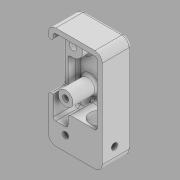
# Autodesk Inventor part: case
Saved by Autodesk Inventor 2020 (Build 240168000, 168)
## iProperties
Created: 2019-10-12
Part Number: case
Material: Generic
Document SubType Name: Modeling
Designer: ROBERTO
Density: 1 g/cm^3
Appearance: Default
Author: gera
Autodesk Inventor part; units mm, degrees
ref_plane "YZ Plane" through (0, 0, 0) normal (1, 0, 0) x (0, 1, 0)
ref_plane "XZ Plane" through (0, 0, 0) normal (0, 1, 0) x (-1, 0, 0)
ref_plane "XY Plane" through (0, 0, 0) normal (0, 0, 1) x (1, 0, 0)
sketch "Sketch1" plane through (0, 0, 0) normal (0, 0, 1) x (1, 0, 0)
  line L0 (9.525, 16.232681) -> (60.325, 16.232681) construction
  line L1 (9.525, 6.707681) -> (60.325, 6.707681)
  arc A0 (0, 16.232681) -> (9.525, 6.707681) centre (9.525, 16.232681) ccw
  arc A1 (60.325, 6.707681) -> (69.85, 16.232681) centre (60.325, 16.232681) ccw
  line L2 (9.525, 130.532681) -> (60.325, 130.532681) construction
  line L3 (60.325, 140.057681) -> (9.525, 140.057681)
  arc A2 (9.525, 140.057681) -> (0, 130.532681) centre (9.525, 130.532681) ccw
  arc A3 (69.85, 130.532681) -> (60.325, 140.057681) centre (60.325, 130.532681) ccw
  line L4 (69.85, 130.532681) -> (69.85, 16.232681)
  line L5 (0, 130.532681) -> (0, 16.232681)
  line L6 (0, -28.406075) -> (0, 170.436448) construction
  point P0 (0, 0)
  point P1 (34.925, 16.232681)
  point P2 (34.925, 130.532681)
  dimension "d0" = 133.35
  dimension "d1" = 69.85
  dimension "d2" = 9.525
  constraints: 16 end point, 8 point on circle, 8 tangent, 4 centre point, 3 equal radius, 2 midpoint, 2 vertical, 1 collinear, 1 horizontal, 1 point on line
  measures "d0" distance between parallel lines of L1 L3
  measures "d1" distance between parallel lines of L4 L5
  measures "d2" radius of A3
extrude "Extrusion1" add sketch "Sketch1" along normal blind 38.1
sketch "Sketch2" plane through (0, 0, 38.1) normal (0, 0, 1) x (1, 0, 0)
  arc A0 (69.85, 130.532681) -> (60.325, 140.057681) centre (60.325, 130.532681) ccw construction
  line L0 (60.325, 140.057681) -> (9.525, 140.057681) construction
  arc A1 (9.525, 140.057681) -> (0, 130.532681) centre (9.525, 130.532681) ccw construction
  line L1 (0, 130.532681) -> (0, 16.232681) construction
  arc A2 (0, 16.232681) -> (9.525, 6.707681) centre (9.525, 16.232681) ccw construction
  line L2 (9.525, 6.707681) -> (60.325, 6.707681) construction
  arc A3 (60.325, 6.707681) -> (69.85, 16.232681) centre (60.325, 16.232681) ccw construction
  line L3 (69.85, 16.232681) -> (69.85, 130.532681) construction
  arc A4 (9.525, 133.707681) -> (6.35, 130.532681) centre (9.525, 130.532681) ccw
  arc A5 (63.5, 130.532681) -> (60.325, 133.707681) centre (60.325, 130.532681) ccw
  arc A6 (60.325, 51.157681) -> (63.5, 54.332681) centre (60.325, 54.332681) ccw
  arc A7 (22.225, 35.282681) -> (25.4, 38.457681) centre (22.225, 38.457681) ccw
  arc A8 (6.35, 38.457681) -> (9.525, 35.282681) centre (9.525, 38.457681) ccw
  line L4 (9.525, 133.707681) -> (61.946324, 133.707681)
  line L5 (6.35, 132.10409) -> (6.35, 35.282681)
  line L6 (63.5, 133.707681) -> (63.5, 54.332681)
  line L7 (69.85, 16.232681) -> (69.85, 130.532681)
  line L8 (6.35, 35.282681) -> (22.225, 35.282681)
  line L9 (25.4, 38.457681) -> (25.4, 50.542115)
  line L10 (60.325, 51.157681) -> (28.575, 51.157681)
  arc A9 (28.575, 51.157681) -> (25.4, 47.982681) centre (28.575, 47.982681) ccw
  point P0 (0, 0)
  dimension "d5" = 6.35
  dimension "d6" = 6.35
  dimension "d7" = 38.1
  dimension "d8" = 15.875
  dimension "d9" = 44.45
  constraints: 12 end point, 12 point on circle, 11 tangent, 6 centre point, 6 point on line, 5 equal radius, 2 coincident, 2 horizontal, 2 vertical, 1 parallel, 1 perpendicular
  measures "d5" distance between parallel lines of L0 L4
  measures "d6" distance between parallel lines of L5 L1
  measures "d7" distance between parallel lines of L6 L9
  measures "d8" distance between parallel lines of L10 L8
  measures "d9" distance between parallel lines of L2 L10
extrude "Extrusion2" cut sketch "Sketch2" against normal blind 31.75 contours L4 A5 L6 A6 L10 A9 L9 A7 L8 A8 L5 A4
sketch "Sketch3" plane through (0, 16.232681, 0) normal (-1, 0, 0) x (0, 0, 1)
  line L0 (0, 114.3) -> (0, 0) construction
  line L1 (0, 0) -> (38.1, 0) construction
  line L2 (38.1, 114.3) -> (38.1, 0) construction
  line L3 (0, 114.3) -> (38.1, 114.3) construction
  line L4 (38.1, 107.95) -> (20.6375, 107.95)
  line L5 (19.05, 106.3625) -> (19.05, 49.2125)
  line L6 (20.6375, 47.625) -> (38.1, 47.625)
  line L7 (38.1, 47.625) -> (38.1, 107.95)
  arc A0 (20.6375, 107.95) -> (19.05, 106.3625) centre (20.6375, 106.3625) ccw
  arc A1 (19.05, 49.2125) -> (20.6375, 47.625) centre (20.6375, 49.2125) ccw
  line L8 (0, 123.825) -> (38.1, 123.825) projected
  point P0 (0, -16.232681)
  dimension "d12" = 19.05
  dimension "d13" = 60.325
  dimension "d14" = 15.875
  dimension "d15" = 3.175
  constraints: 8 end point, 4 point on circle, 4 tangent, 2 centre point, 2 parallel, 1 collinear, 1 equal radius, 1 horizontal, 1 perpendicular
  measures "d12" distance between parallel lines of L5 L2
  measures "d13" distance between parallel lines of L6 L4
  measures "d14" distance between parallel lines of L4 L8
  measures "d15" diameter of A0
extrude "Extrusion3" cut sketch "Sketch3" against normal blind 6.35
sketch "Sketch4" plane through (0, 0, 6.35) normal (0, 0, 1) x (1, 0, 0)
  line L0 (25.4, 47.982681) -> (25.4, 38.457681) construction
  arc A0 (28.575, 51.157681) -> (25.4, 47.982681) centre (28.575, 47.982681) ccw construction
  line L1 (60.325, 51.157681) -> (28.575, 51.157681) construction
  arc A1 (60.325, 51.157681) -> (63.5, 54.332681) centre (60.325, 54.332681) ccw construction
  line L2 (63.5, 130.532681) -> (63.5, 54.332681) construction
  arc A2 (63.5, 130.532681) -> (60.325, 133.707681) centre (60.325, 130.532681) ccw construction
  line L3 (9.525, 133.707681) -> (60.325, 133.707681) construction
  arc A3 (9.525, 133.707681) -> (6.35, 130.532681) centre (9.525, 130.532681) ccw construction
  line L4 (6.35, 38.457681) -> (6.35, 130.532681) construction
  arc A4 (6.35, 38.457681) -> (9.525, 35.282681) centre (9.525, 38.457681) ccw construction
  line L5 (22.225, 35.282681) -> (9.525, 35.282681) construction
  arc A5 (22.225, 35.282681) -> (25.4, 38.457681) centre (22.225, 38.457681) ccw construction
  line L6 (0, 65.445181) -> (0, 122.595181) construction
  line L7 (0, 65.445181) -> (0, 122.595181) construction
  line L8 (0, 65.445181) -> (6.35, 65.445181) construction
  line L9 (6.35, 122.595181) -> (6.35, 65.445181) construction
  line L10 (0, 122.595181) -> (6.35, 122.595181) construction
  line L11 (6.35, 63.857681) -> (0, 63.857681) construction
  line L12 (0, 63.857681) -> (0, 16.232681) construction
  arc A6 (0, 16.232681) -> (9.525, 6.707681) centre (9.525, 16.232681) ccw construction
  line L13 (9.525, 6.707681) -> (60.325, 6.707681) construction
  arc A7 (60.325, 6.707681) -> (69.85, 16.232681) centre (60.325, 16.232681) ccw construction
  line L14 (69.85, 16.232681) -> (69.85, 130.532681) construction
  arc A8 (69.85, 130.532681) -> (60.325, 140.057681) centre (60.325, 130.532681) ccw construction
  line L15 (60.325, 140.057681) -> (9.525, 140.057681) construction
  arc A9 (9.525, 140.057681) -> (0, 130.532681) centre (9.525, 130.532681) ccw construction
  line L16 (0, 130.532681) -> (0, 124.182681) construction
  line L17 (0, 124.182681) -> (6.35, 124.182681) construction
  line L18 (6.35, 124.182681) -> (6.35, 130.532681) construction
  arc A10 (9.525, 133.707681) -> (6.35, 130.532681) centre (9.525, 130.532681) ccw construction
  line L19 (9.525, 133.707681) -> (60.325, 133.707681) construction
  arc A11 (63.5, 130.532681) -> (60.325, 133.707681) centre (60.325, 130.532681) ccw construction
  line L20 (63.5, 130.532681) -> (63.5, 54.332681) construction
  arc A12 (60.325, 51.157681) -> (63.5, 54.332681) centre (60.325, 54.332681) ccw construction
  line L21 (60.325, 51.157681) -> (28.575, 51.157681) construction
  arc A13 (28.575, 51.157681) -> (25.4, 47.982681) centre (28.575, 47.982681) ccw construction
  line L22 (25.4, 47.982681) -> (25.4, 38.457681) construction
  arc A14 (22.225, 35.282681) -> (25.4, 38.457681) centre (22.225, 38.457681) ccw construction
  line L23 (22.225, 35.282681) -> (9.525, 35.282681) construction
  arc A15 (6.35, 38.457681) -> (9.525, 35.282681) centre (9.525, 38.457681) ccw construction
  line L24 (6.35, 38.457681) -> (6.35, 63.857681) construction
  line L25 (0, 124.182681) -> (6.35, 124.182681)
  line L26 (6.35, 124.182681) -> (12.7, 124.182681)
  line L27 (12.7, 98.782681) -> (6.35, 98.782681)
  line L28 (6.35, 124.182681) -> (6.35, 98.782681)
  line L29 (6.35, 38.457681) -> (6.35, 130.532681)
  arc A16 (6.35, 122.481204) -> (5.46153, 121.917936) centre (12.7, 111.482681) ccw
  arc A17 (12.7, 98.782681) -> (12.7, 124.182681) centre (12.7, 111.482681) ccw
  point P0 (0, 0)
  dimension "d19" = 104.775
  dimension "d20" = 12.7
  constraints: 6 end point, 5 point on circle, 2 centre point, 2 point on line, 1 horizontal, 1 tangent, 3 other
  measures "d19" distance from line of L13 A16.centre
  measures "d20" distance from line of A16.centre L6
extrude "Extrusion4" add sketch "Sketch4" along normal blind 12.7
sketch "Sketch5" plane through (0, 0, 6.35) normal (0, 0, 1) x (1, 0, 0)
  circle A0 centre (22.225, 67.032681) radius 9.525
  line L0 (6.35, 63.857681) -> (0, 63.857681) construction
  line L1 (0, 63.857681) -> (0, 16.232681) construction
  arc A1 (0, 16.232681) -> (9.525, 6.707681) centre (9.525, 16.232681) ccw construction
  line L2 (9.525, 6.707681) -> (60.325, 6.707681) construction
  arc A2 (60.325, 6.707681) -> (69.85, 16.232681) centre (60.325, 16.232681) ccw construction
  line L3 (69.85, 16.232681) -> (69.85, 130.532681) construction
  arc A3 (69.85, 130.532681) -> (60.325, 140.057681) centre (60.325, 130.532681) ccw construction
  line L4 (60.325, 140.057681) -> (9.525, 140.057681) construction
  arc A4 (9.525, 140.057681) -> (0, 130.532681) centre (9.525, 130.532681) ccw construction
  line L5 (0, 130.532681) -> (0, 124.182681) construction
  line L6 (0, 124.182681) -> (6.35, 124.182681) construction
  line L7 (6.35, 124.182681) -> (6.35, 130.532681) construction
  arc A5 (9.525, 133.707681) -> (6.35, 130.532681) centre (9.525, 130.532681) ccw construction
  line L8 (9.525, 133.707681) -> (60.325, 133.707681) construction
  arc A6 (63.5, 130.532681) -> (60.325, 133.707681) centre (60.325, 130.532681) ccw construction
  line L9 (63.5, 130.532681) -> (63.5, 54.332681) construction
  arc A7 (60.325, 51.157681) -> (63.5, 54.332681) centre (60.325, 54.332681) ccw construction
  line L10 (60.325, 51.157681) -> (28.575, 51.157681) construction
  arc A8 (28.575, 51.157681) -> (25.4, 47.982681) centre (28.575, 47.982681) ccw construction
  line L11 (25.4, 47.982681) -> (25.4, 38.457681) construction
  arc A9 (22.225, 35.282681) -> (25.4, 38.457681) centre (22.225, 38.457681) ccw construction
  line L12 (22.225, 35.282681) -> (9.525, 35.282681) construction
  arc A10 (6.35, 38.457681) -> (9.525, 35.282681) centre (9.525, 38.457681) ccw construction
  line L13 (6.35, 38.457681) -> (6.35, 63.857681) construction
  line L14 (6.35, 124.182681) -> (12.7, 124.182681) construction
  arc A11 (12.7, 98.782681) -> (12.7, 124.182681) centre (12.7, 111.482681) ccw construction
  line L15 (12.7, 98.782681) -> (6.35, 98.782681) construction
  line L16 (6.35, 38.457681) -> (6.35, 98.782681) construction
  arc A12 (6.35, 38.457681) -> (9.525, 35.282681) centre (9.525, 38.457681) ccw construction
  line L17 (22.225, 35.282681) -> (9.525, 35.282681) construction
  arc A13 (22.225, 35.282681) -> (25.4, 38.457681) centre (22.225, 38.457681) ccw construction
  line L18 (25.4, 47.982681) -> (25.4, 38.457681) construction
  arc A14 (28.575, 51.157681) -> (25.4, 47.982681) centre (28.575, 47.982681) ccw construction
  line L19 (60.325, 51.157681) -> (28.575, 51.157681) construction
  arc A15 (60.325, 51.157681) -> (63.5, 54.332681) centre (60.325, 54.332681) ccw construction
  line L20 (63.5, 130.532681) -> (63.5, 54.332681) construction
  arc A16 (63.5, 130.532681) -> (60.325, 133.707681) centre (60.325, 130.532681) ccw construction
  line L21 (9.525, 133.707681) -> (60.325, 133.707681) construction
  arc A17 (9.525, 133.707681) -> (6.35, 130.532681) centre (9.525, 130.532681) ccw construction
  line L22 (6.35, 124.182681) -> (6.35, 130.532681) construction
  point P0 (0, 0)
  dimension "d25" = 19.05
  dimension "d26" = 60.325
  dimension "d27" = 22.225
  constraints: 1 centre point
  measures "d25" diameter of A0
  measures "d26" distance from line of L2 A0.centre
  measures "d27" distance from line of L1 A0.centre
extrude "Extrusion5" add sketch "Sketch5" along normal blind 31.75
sketch "Sketch6" plane through (9.525, 6.707681, 0) normal (0, -1, 0) x (1, 0, 0)
  line L0 (60.325, 0) -> (60.325, 38.1) construction
  line L1 (0, 38.1) -> (50.8, 38.1) construction
  point P0 (-9.525, 0)
  point P1 (41.275, 22.225)
  dimension "d30" = 19.05
  dimension "d31" = 15.875
  measures "d30" distance from line of L0 point (41.275, 22.225)
  measures "d31" distance from line of L1 point (41.275, 22.225)
hole "Hole1" at (50.8, 6.707681, 22.225) direction (0, 1, 0) diameter 25.4 depth 44.45 tip angle 118
fillet "Fillet1" radius 3.175 15 edges at (12.7, 67.0327, 6.35) (7.2799, 36.2126, 6.35) (15.875, 35.2827, 6.35) (24.4701, 36.2126, 6.35) (25.4, 43.2202, 6.35) (26.3299, 50.2277, 6.35) (44.45, 51.1577, 6.35) (62.5701, 52.0876, 6.35) (63.5, 92.4327, 6.35) (62.5701, 132.7777, 6.35) (34.925, 133.7077, 6.35) (7.2799, 132.7777, 6.35) (6.35, 127.3577, 6.35) (6.35, 68.6202, 6.35) (6.35, 124.1827, 12.7)
fillet "Fillet2" radius 3.175 6 edges at (11.1124, 98.7827, 6.35) (7.2799, 98.7827, 7.2799) (6.35, 98.7827, 14.2875) (11.1124, 124.1827, 6.35) (7.2799, 125.1126, 7.2799) (25.4, 111.4827, 6.35)
fillet "Fillet3" radius 3.175 7 edges at (0, 64.3226, 19.515) (0, 94.0202, 19.05) (0, 123.7177, 19.515) (0, 124.1827, 29.3687) (0, 63.8577, 29.3688) (6.35, 124.1827, 29.3687) (6.35, 123.7177, 19.515)
fillet "Fillet4" radius 3.175 8 edges at (67.0602, 9.4975, 0) (69.85, 73.3827, 0) (67.0602, 137.2679, 0) (34.925, 140.0577, 0) (2.7898, 137.2679, 0) (0, 73.3827, 0) (2.7898, 9.4975, 0) (34.925, 6.7077, 0)
sketch "Sketch7" plane through (12.7, 111.482681, 19.05) normal (0, 0, 1) x (1, 0, 0)
  line L0 (-9.525, -46.0375) -> (-9.525, 11.1125) construction
  line L1 (-9.525, -46.0375) -> (-6.35, -46.0375) construction
  line L2 (-6.35, -15.875) -> (-6.35, -46.0375) construction
  arc A0 (-3.175, -12.7) -> (-6.35, -15.875) centre (-3.175, -15.875) ccw construction
  line L3 (-3.175, -12.7) -> (0, -12.7) construction
  arc A1 (0, -12.7) -> (0, 12.7) centre (0, 0) ccw construction
  line L4 (0, 12.7) -> (-3.175, 12.7) construction
  arc A2 (-6.35, 15.875) -> (-3.175, 12.7) centre (-3.175, 15.875) ccw construction
  line L5 (-6.35, 15.602628) -> (-6.35, 15.875) construction
  arc A3 (0, -12.7) -> (0, 12.7) centre (0, 0) ccw construction
  point P0 (-12.7, -111.482681)
  constraints: 1 coincident, 1 other
hole "Hole2" at (12.7, 111.482681, 19.05) direction (0, 0, -1) diameter 9.525 end through all
sketch "Sketch11" plane through (69.85, 16.232681, 38.1) normal (1, 0, 0) x (0, 0, -1)
  line L0 (0, 0) -> (0, 114.3)
  line L1 (34.925, -9.525) -> (24.27526, -9.525)
  point P0 (38.1, -16.232681)
  point P1 (15.875, 12.7)
  dimension "d75" = 15.875
  dimension "d76" = 22.225
  measures "d75" distance from line of L0 point (15.875, 12.7)
  measures "d76" distance from line of L1 point (15.875, 12.7)
hole "Hole6" at (69.85, 28.932681, 22.225) direction (-1, 0, 0) diameter 7.9375 depth 15.24
sketch "Sketch12" plane through (0, 0, 0) normal (0, 0, -1) x (-1, 0, 0)
  line L0 (0, 16.232681) -> (0, 130.532681)
  line L1 (-60.325, 6.707681) -> (-9.525, 6.707681)
  point P0 (0, 0)
  point P1 (-22.225, 67.032681)
  dimension "d86" = 22.225
  dimension "d87" = 60.325
  measures "d86" distance from line of L0 point (-22.225, 67.033)
  measures "d87" distance from line of L1 point (-22.225, 67.033)
hole "Hole7" at (22.225, 67.032681, 0) direction (0, 0, 1) diameter 7.9375 end through all counterbore diameter 12.7 counterbore depth 7.9375
sketch "Sketch13" plane through (0, 0, 0) normal (0, 0, -1) x (-1, 0, 0)
  line L0 (0, 16.232681) -> (0, 130.532681)
  line L1 (-60.325, 6.707681) -> (-9.525, 6.707681)
  point P0 (0, 0)
  point P1 (-22.225, 25.757681)
  dimension "d95" = 22.225
  dimension "d96" = 19.05
  measures "d95" distance from line of L0 point (-22.225, 25.758)
  measures "d96" distance from line of L1 point (-22.225, 25.758)
hole "Hole8" at (22.225, 25.757681, 0) direction (0, 0, 1) diameter 7.9375 end through all counterbore diameter 12.7 counterbore depth 7.9375
body "Solid1"
